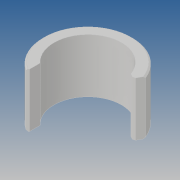
# Autodesk Inventor part: viseur_base
Saved by Autodesk Inventor 2019 (Build 230136000, 136)
## iProperties
Created: 2019-01-06
Part Number: viseur_base
Material: Générique
Document SubType Name: Modeling
Designer: Theo
Density: 1 g/cm^3
Appearance: Par défaut
Author: Theo
Autodesk Inventor part; units mm, degrees
ref_plane "YZ Plane" through (0, 0, 0) normal (1, 0, 0) x (0, 1, 0)
ref_plane "XZ Plane" through (0, 0, 0) normal (0, 1, 0) x (-1, 0, 0)
ref_plane "XY Plane" through (0, 0, 0) normal (0, 0, 1) x (1, 0, 0)
sketch "Esquisse1" plane through (0, 0, 0) normal (0, 1, 0) x (-1, 0, 0)
  arc A0 (-8.5, 9.1652) -> (8.5, 9.1652) centre (0, 0) ccw
  line L0 (8.5, 9.1652) -> (8.5, 14.1652)
  line L1 (-8.5, 9.1652) -> (-8.5, 14.1652)
  arc A1 (-8.5, 14.1652) -> (8.5, 14.1652) centre (0, 0) ccw
  line L2 (-12.0741, -3.2352) -> (-15.9568, -4.2756)
  line L3 (23.1276, 0) -> (-23.1276, 0) projected
  point P0 (-14.1537, -8.5191)
  dimension "d0" = 12.5
  dimension "d1" = 5
  dimension "d2" = 17
  dimension "d11" = 15
  constraints: 7 point on circle, 6 end point, 2 centre point, 2 coincident, 2 vertical, 1 horizontal alignment, 1 line through centre, 1 parallel
  measures "d0" radius of A0
  measures "d1" distance of L1.start L1.end
  measures "d2" distance between parallel lines of L0 L1
  measures "d11" angle of L3 L2
extrude "Extrusion1" add sketch "Esquisse1" along normal mid plane 20 contours A0 L3 A1 L2 | A0 L0 A1 L3 picked at (15.0221, -1.3088)
chamfer "Chanfrein1" distance 1 angle 45 2 edges at (-8.5, 0, 14.1652) (12.0741, 0, -3.2352)
chamfer "Chanfrein2" distance 0.5 angle 45 2 edges at (-9.5419, 10, -13.4853) (-9.5419, -10, -13.4853)
chamfer "Chanfrein3" distance 2 angle 45 1 edges at (15.9568, 0, -4.2756)
